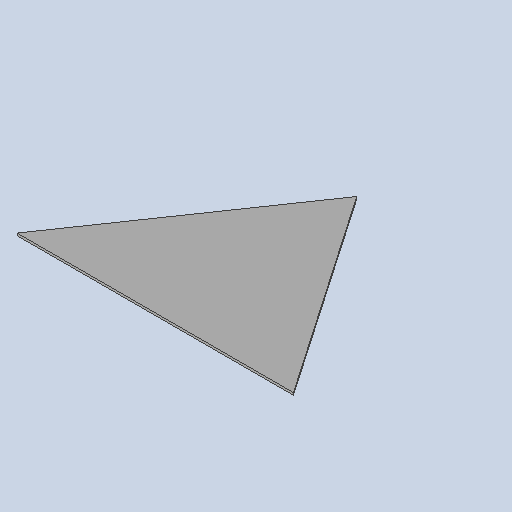
# Autodesk Inventor part: MSC 103 ROСKET NOSE
Saved by Autodesk Inventor 2025 (Build 290162010, 162A)
## iProperties
Created: 2024-05-19
Part Number: MSC 103 ROСKET NOSE
Material: Stainless Steel
Document SubType Name: Sheet Metal
Designer: admin
Density: 8 g/cm^3
Sheet Metal Rule: AISI304 2mm Die16
Sheet Metal Width: 175,000 mm
Sheet Metal Length: 240,000 mm
Sheet Metal Area: 42000,000 mm^2
Appearance: Default
Stock Number: МОО 103 ракета нос
Mass: 336 g
Surface Area: 433.288 cm^2
Volume: 42 cm^3
Flat Pattern Width: 17.5 cm
Flat Pattern Length: 24 cm
Flat Pattern Area: 420 cm^2
Author: admin
Autodesk Inventor part; units mm, degrees
ref_plane "YZ Plane" through (0, 0, 0) normal (1, 0, 0) x (0, 1, 0)
ref_plane "XZ Plane" through (0, 0, 0) normal (0, 1, 0) x (-1, 0, 0)
ref_plane "XY Plane" through (0, 0, 0) normal (0, 0, 1) x (1, 0, 0)
sketch "Sketch2" plane through (0, 0, 0) normal (0, 0, 1) x (1, 0, 0)
  line L0 (120, 0) -> (-120, 0)
  line L1 (-120, 0) -> (0, 175)
  line L2 (0, 175) -> (120, 0)
  point P0 (0, 0)
  point P1 (0, 0)
  dimension "d8" = 240
  dimension "d9" = 175
  measures "d8" distance of L0.start L0.end
  measures "d9" distance of L1.end point (0, 0)
extrude "Plate1" add sketch "Sketch2" along normal blind 2
equation "\"d7\" = Thickness"
equation "\"BendReliefWidth\" = Thickness"
equation "\"BendReliefDepth\" = 0.5 * Thickness"
equation "\"CornerReliefSize\" = 4 * Thickness"
equation "\"MinimumRemnant\" = 2 * Thickness"
equation "\"TransitionRadius\" = BendRadius"
equation "\"JacobiRadiusSize\" = BendRadius"
equation "\"GapSize\" = Thickness"
equation "\"Thickness\" = 2"
equation "\"BendRadius\" = 2.75"
body "Solid2"
